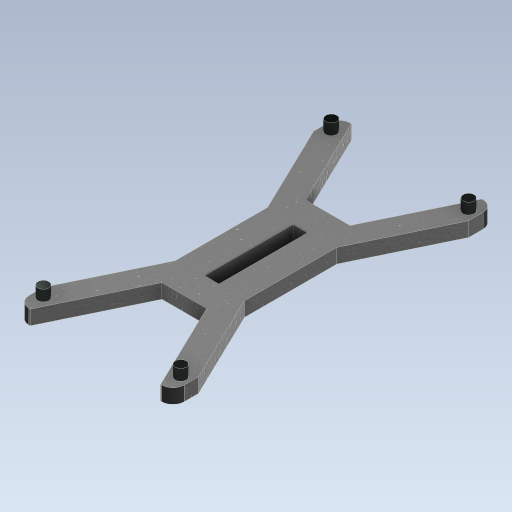
# Autodesk Inventor part: SoportePlaca
Saved by Autodesk Inventor 2023 (Build 270158000, 158)
## iProperties
Created: 2023-03-18
Part Number: SoportePlaca
Material: Rubber, Silicone
Document SubType Name: Modeling
Designer: santi
Density: 1.25 g/cm^3
Appearance: Rubber - Black
Author: santi
Autodesk Inventor part; units mm, degrees
ref_plane "YZ Plane" through (0, 0, 0) normal (1, 0, 0) x (0, 1, 0)
ref_plane "XZ Plane" through (0, 0, 0) normal (0, 1, 0) x (-1, 0, 0)
ref_plane "XY Plane" through (0, 0, 0) normal (0, 0, 1) x (1, 0, 0)
sketch "Sketch1" plane through (0, 0, 0) normal (0, 1, 0) x (-1, 0, 0)
  line L0 (0, 0) -> (140, 0) construction
  line L1 (140, 0) -> (140, -290) construction
  line L2 (140, -290) -> (0, -290) construction
  line L3 (0, -290) -> (0, 0) construction
  line L4 (0, 0) -> (140, -290) construction
  line L5 (11.1043, 0) -> (140, -266.9982) construction
  line L6 (0, -23.0018) -> (128.8957, -290) construction
  line L7 (-10, -2.2875) -> (-10, 0)
  line L8 (140, 0) -> (0, -290) construction
  line L9 (140, -23.0018) -> (11.1043, -290) construction
  line L10 (128.8957, 0) -> (0, -266.9982) construction
  line L11 (150, -2.2875) -> (150, 0)
  line L12 (0, -23.0018) -> (0, 0)
  line L13 (140, -23.0018) -> (140, 0)
  line L14 (140, -266.9982) -> (140, -290)
  line L15 (0, -266.9982) -> (0, -290)
  line L16 (76.5, -105) -> (63.5, -105) construction
  line L17 (63.5, -105) -> (63.5, -185) construction
  line L18 (63.5, -185) -> (76.5, -185) construction
  line L19 (76.5, -185) -> (76.5, -105) construction
  line L20 (101.2667, -80.2333) -> (38.7333, -80.2333) construction
  line L21 (38.7333, -80.2333) -> (38.7333, -209.7667) construction
  line L22 (38.7333, -209.7667) -> (101.2667, -209.7667) construction
  line L23 (101.2667, -209.7667) -> (101.2667, -80.2333) construction
  line L24 (0, -23.0018) -> (38.7333, -103.2351)
  line L25 (38.7333, -186.7649) -> (0, -266.9982)
  line L26 (0, -290) -> (11.1043, -290)
  line L27 (49.8376, -209.7667) -> (90.1624, -209.7667)
  line L28 (49.8376, -209.7667) -> (11.1043, -290)
  line L29 (38.7333, -103.2351) -> (38.7333, -186.7649)
  line L30 (90.1624, -209.7667) -> (128.8957, -290)
  line L31 (128.8957, -290) -> (140, -290)
  line L32 (140, -266.9982) -> (101.2667, -186.7649)
  line L33 (101.2667, -186.7649) -> (101.2667, -103.2351)
  line L34 (101.2667, -103.2351) -> (140, -23.0018)
  line L35 (128.8957, 0) -> (90.1624, -80.2333)
  line L36 (90.1624, -80.2333) -> (49.8376, -80.2333)
  line L37 (49.8376, -80.2333) -> (11.1043, 0)
  line L38 (11.1043, 0) -> (0, 0)
  line L39 (128.8957, 0) -> (140, 0)
  line L40 (63.5, -105) -> (76.5, -105)
  line L41 (76.5, -185) -> (63.5, -185)
  line L42 (63.5, -105) -> (63.5, -185)
  line L43 (76.5, -185) -> (76.5, -105)
  point P0 (70, -105)
  point P1 (70, 0)
  point P2 (140, -145)
  point P3 (76.5, -145)
  dimension "d0" = 140
  dimension "d1" = 290
  dimension "d2" = 10
  dimension "d3" = 10
  dimension "d4" = 10
  dimension "d5" = 10
  dimension "d6" = 13
  dimension "d7" = 80
  constraints: 88 end point, 29 point on line, 13 collinear, 8 parallel, 4 midpoint, 4 perpendicular, 2 horizontal, 1 horizontal alignment, 1 vertical alignment, 3 other
  measures "d0" distance of L1.end L2.end
  measures "d1" distance of L0.end L1.end
  measures "d2" distance between parallel lines of L4 L5
  measures "d3" distance between parallel lines of L4 L6
  measures "d4" distance between parallel lines of L8 L9
  measures "d5" distance between parallel lines of L8 L10
  measures "d6" distance of L18.end L17.end
  measures "d7" distance of L17.end L16.end
extrude "Extrusion1" add sketch "Sketch1" along normal blind 13
fillet "Fillet1" radius 10 4 edges at (-140, 6.5, -290) (0, 6.5, -290) (0, 6.5, 0) (-140, 6.5, 0)
sketch "Sketch2" plane through (0, 13, 0) normal (0, 1, 0) x (1, 0, 0)
  circle A0 centre (-8, 275) radius 5
  line L0 (-10, 290) -> (-11.1043, 290) projected
  line L1 (0, 266.9982) -> (0, 280) construction
  line L2 (-70, 345.1807) -> (-70, -192.6697) construction
  line L3 (0, 10) -> (0, 23.0018) construction
  line L4 (-90.1624, 80.2333) -> (-49.8376, 80.2333) construction
  circle A1 centre (-132, 275) radius 5
  line L5 (-255.5862, 145) -> (85.936, 145)
  line L6 (-38.7333, 103.2351) -> (-38.7333, 186.7649) construction
  circle A2 centre (-8, 15) radius 5
  circle A3 centre (-132, 15) radius 5
  point P0 (0, 0)
  point P1 (-70, 80.2333)
  point P2 (-38.7333, 145)
  dimension "d11" = 10
  dimension "d12" = 15
  dimension "d13" = 8
  dimension "d14" = 537.8504
  dimension "d15" = 341.5222
  constraints: 4 centre point, 4 end point, 3 symmetric about line, 2 midpoint, 2 point on line, 1 horizontal, 1 parallel, 3 other
  measures "d11" diameter of A0
  measures "d12" distance from line of L0 A0.centre
  measures "d13" distance from line of L1 A0.centre
  measures "d14" distance of L2.start L2.end
  measures "d15" distance of L5.start L5.end
extrude "Extrusion2" add sketch "Sketch2" along normal blind 10
body "Solid1"
